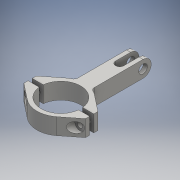
# Autodesk Inventor part: Potentiometer arm
Saved by Autodesk Inventor 2016 (Build 200138000, 138)
## iProperties
Created: 2017-03-29
Part Number: Potentiometer arm
Material: Generic
Document SubType Name: Modeling
Designer: BenjaPad
Density: 1 g/cm^3
Appearance: Default
Author: BenjaPad
Autodesk Inventor part; units mm, degrees
ref_plane "YZ Plane" through (0, 0, 0) normal (1, 0, 0) x (0, 1, 0)
sketch "Sketch1" plane through (0, 0, 0) normal (0, 0, 1) x (1, 0, 0)
  circle A0 centre (0, 0) radius 9.65
  circle A1 centre (0, 0) radius 11.65
  line L0 (15, -3) -> (15, 3)
  line L1 (-15, 3) -> (-15, -3)
  line L2 (-15, -3) -> (15, 3) construction
  line L3 (15, -3) -> (-15, 3) construction
  line L4 (-15, -3) -> (-9.1718, -3)
  line L5 (9.1718, -3) -> (15, -3)
  line L6 (15, 3) -> (9.1718, 3)
  line L7 (-9.1718, 3) -> (-15, 3)
  dimension "d0" = 19.3
  dimension "d1" = 2
  dimension "d2" = 30
  dimension "d3" = 6
  constraints: 16 end point, 5 parallel, 4 point on circle, 2 centre point, 2 horizontal, 2 midpoint, 2 perpendicular, 1 coincident
  measures "d0" diameter of A0
  measures "d1" radial gap between concentric circles of A0 A1
  measures "d2" distance of L1.start L0.end
  measures "d3" distance of L0.end L0.start
extrude "Extrusion1" add sketch "Sketch1" along normal blind 8 contours A0 L6 A1 L5 | A0 L7 A1 L6 | L5 A1 L4 A0 | A0 L4 A1 L7 | L6 L0 L5 A1 | A1 L4 L1 L7
sketch "Sketch2" plane through (0, 0, 8) normal (0, 0, 1) x (1, 0, 0)
  line L0 (-15, 3) -> (-15, -3) projected
  line L1 (-15, 3) -> (-7.2195, 9.1434)
  line L2 (15, 3) -> (11.2571, 3) projected
  line L3 (7.2195, 9.1434) -> (15, 3)
  line L4 (-15, -3) -> (-11.2571, -3) projected
  line L5 (-7.2195, -9.1434) -> (-15, -3)
  arc A0 (11.2571, 3) -> (-11.2571, 3) centre (0, 0) ccw projected
  arc A1 (-11.2571, -3) -> (11.2571, -3) centre (0, 0) ccw projected
  line L6 (11.2571, -3) -> (15, -3) projected
  line L7 (15, -3) -> (7.2195, -9.1434)
  line L8 (-11.2571, 3) -> (-15, 3) projected
  constraints: 8 end point, 4 point on circle, 4 tangent
extrude "Extrusion2" add sketch "Sketch2" against normal blind 8
sketch "Sketch3" plane through (0, 0, 8) normal (0, 0, 1) x (1, 0, 0)
  line L0 (-24.7008, -1) -> (24.7008, -1)
  line L1 (24.7008, -1) -> (24.7008, 1)
  line L2 (24.7008, 1) -> (-24.7008, 1)
  line L3 (-24.7008, 1) -> (-24.7008, -1)
  line L4 (-24.7008, -1) -> (24.7008, 1) construction
  line L5 (24.7008, -1) -> (-24.7008, 1) construction
  point P0 (0, 0)
  dimension "d8" = 2
  constraints: 12 end point, 2 midpoint, 2 parallel, 1 horizontal, 1 perpendicular
  measures "d8" distance of L1.end L0.end
extrude "Extrusion3" cut sketch "Sketch3" against normal through all
sketch "Sketch4" plane through (0, 0, 0) normal (0, 0, -1) x (-1, 0, 0)
  line L0 (-4, 0) -> (-2, 0)
  line L1 (-2, 11.477) -> (-2, 40)
  line L2 (-2, 40) -> (-4, 40)
  line L3 (-4, 40) -> (-4, 10.9418)
  line L4 (2, 40) -> (4, 40)
  line L5 (4, 40) -> (4, 10.9418)
  line L6 (4, 0) -> (2, 0)
  line L7 (2, 11.477) -> (2, 40)
  arc A0 (7.2195, 9.1434) -> (-7.2195, 9.1434) centre (0, 0) ccw projected
  point P0 (-3, 0)
  dimension "d11" = 2
  dimension "d12" = 2
  dimension "d13" = 4
  dimension "d14" = 2
  dimension "d15" = 40
  constraints: 16 end point, 4 parallel, 4 point on circle, 2 horizontal, 2 perpendicular, 2 point on line, 1 horizontal alignment, 1 midpoint
  measures "d11" distance of L4.start L4.end
  measures "d12" distance of L1.end L2.end
  measures "d13" distance between parallel lines of L1 L7
  measures "d14" distance from line of point (0, 0) L1
  measures "d15" distance from line of point (0, 0) L2
extrude "Extrusion4" add sketch "Sketch4" against normal blind 8
fillet "Fillet1" radius 2 4 edges at (-4, 10.9418, 4) (-2, 11.477, 4) (2, 11.477, 4) (4, 10.9418, 4)
fillet "Fillet2" radius 4 4 edges at (-3, 40, 0) (3, 40, 0) (3, 40, 8) (-3, 40, 8)
ref_plane "Work Plane1" through (-15, -3, 8) normal (0, 1, 0) x (1, 0, 0)
sketch "Sketch5" plane through (-15, -3, 8) normal (0, 1, 0) x (1, 0, 0)
  line L0 (0, 8) -> (5.402, 8) projected
  line L1 (0, 0) -> (0, 8) projected
  circle A0 centre (2.701, 4) radius 2.5
  point P0 (15, 8)
  dimension "d21" = 5
  constraints: 1 centre point
  measures "d21" diameter of A0
extrude "Extrusion5" cut sketch "Sketch5" against normal blind 8
sketch "Sketch6" plane through (-12.299, -3, 4) normal (0, -1, 0) x (1, 0, 0)
  circle A0 centre (0, 0) radius 1.25
  point P0 (12.299, -4)
  dimension "d24" = 2.5
  constraints: 1 centre point
  measures "d24" diameter of A0
extrude "Extrusion6" cut sketch "Sketch6" against normal blind 12
ref_plane "Work Plane2" through (-15, 3, 8) normal (0, -1, 0) x (1, 0, 0)
sketch "Sketch7" plane through (-15, 3, 8) normal (0, -1, 0) x (1, 0, 0)
  circle A0 centre (2.701, -4) radius 1.25 projected
  circle A1 centre (2.701, -4) radius 2.5 projected
  point P0 (15, -8)
extrude "Extrusion7" cut sketch "Sketch7" against normal blind 12
mirror "Mirror1" about plane through (0, 0, 0) normal (1, 0, 0) of "Extrusion7", "Extrusion6", "Extrusion5"
sketch "Sketch8" plane through (-4, 12.2606, 0) normal (-1, 0, 0) x (0, 0, 1)
  arc A0 (8, 23.7394) -> (0, 23.7394) centre (4, 23.7394) ccw projected
  line L0 (0, 0) -> (0, 23.7394) projected
  line L1 (8, 0) -> (0, 0) projected
  line L2 (8, 23.7394) -> (8, 0) projected
  circle A1 centre (4, 23.7394) radius 2.1
  point P0 (0, -12.2606)
  dimension "d30" = 4.2
  constraints: 1 centre point, 1 coincident
  measures "d30" diameter of A1
extrude "Extrusion8" cut sketch "Sketch8" against normal through all contours A1
sketch "Sketch9" plane through (0, 0, 8) normal (0, 0, 1) x (1, 0, 0)
  line L0 (-4, 36) -> (-2, 36) projected
  line L1 (-4, 36) -> (-4, 12.2606) projected
  arc A0 (-5.1209, 10.4642) -> (-4, 12.2606) centre (-6, 12.2606) ccw projected
  arc A1 (-5.1209, 10.4642) -> (-7.2195, 9.1434) centre (0, 0) ccw projected
  line L2 (-7.2195, 9.1434) -> (-15, 3) projected
  line L3 (-15, 3) -> (-15, 1) projected
  line L4 (-15, 1) -> (-9.598, 1) projected
  arc A2 (9.598, 1) -> (-9.598, 1) centre (0, 0) ccw projected
  line L5 (9.598, 1) -> (15, 1) projected
  line L6 (15, 1) -> (15, 3) projected
  line L7 (15, 3) -> (7.2195, 9.1434) projected
  arc A3 (7.2195, 9.1434) -> (5.1209, 10.4642) centre (0, 0) ccw projected
  arc A4 (4, 12.2606) -> (5.1209, 10.4642) centre (6, 12.2606) ccw projected
  line L8 (4, 12.2606) -> (4, 36) projected
  line L9 (2, 36) -> (4, 36) projected
  line L10 (2, 36) -> (2, 13.65) projected
  arc A5 (-2, 13.65) -> (2, 13.65) centre (0, 13.65) ccw projected
  line L11 (-2, 13.65) -> (-2, 36) projected
  arc A6 (-2, 28.65) -> (2, 28.65) centre (0, 28.65) ccw
  line L12 (2, 36) -> (2, 13.65) projected
  dimension "d33" = 15
  constraints: 2 point on circle, 2 point on line, 2 tangent, 1 centre point
  measures "d33" distance of A5.centre A6.centre
extrude "Extrusion9" add sketch "Sketch9" against normal blind 8 contours A6 L10 A5 L11
body "Solid1"
